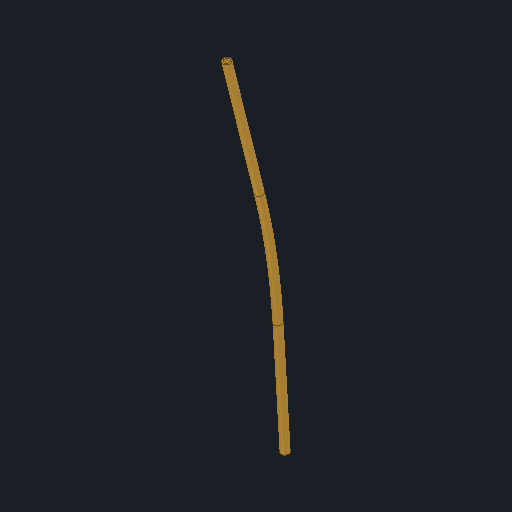
# Autodesk Inventor part: prop_shaft
Saved by Autodesk Inventor 2023 (Build 270158030, 158C)
## iProperties
Created: 2022-04-18
Part Number: prop_shaft
Material: Generic
Document SubType Name: Modeling
Designer: kardo
Density: 1 g/cm^3
Appearance: Brass - Prop shaft
Author: kardo
Autodesk Inventor part; units mm, degrees
ref_plane "YZ Plane" through (0, 0, 0) normal (1, 0, 0) x (0, 1, 0)
ref_plane "XZ Plane" through (0, 0, 0) normal (0, 1, 0) x (-1, 0, 0)
ref_plane "XY Plane" through (0, 0, 0) normal (0, 0, 1) x (1, 0, 0)
derived "stencil_frame.ipt"
sketch "sk_drivetrain_profile" plane through (6, 0, 0) normal (1, 0, 0) x (0, 1, 0)
  line L0 (-547.3485, 0) -> (393.091, 0) construction
  line L1 (-363, 4666.1952) -> (-363, -2045.0469) construction
  line L2 (0, 4666.1952) -> (0, -2045.0469) construction
  line L3 (-140.6277, 54.4571) -> (-133.8539, 27.2888)
  line L4 (-395, 0) -> (-331.1194, 3.9071)
  line L5 (-137.2408, 40.8729) -> (-228.5101, 18.117)
  line L6 (-314.0499, 4.9511) -> (-270.6751, 7.604) construction
  line L7 (-270.6751, 7.604) -> (-228.5101, 18.117) construction
  line L8 (-133.8539, 27.2888) -> (-133.8539, 22.2888) construction
  line L9 (-331.1194, 3.9071) -> (-314.0499, 4.9511)
  line L10 (-1246.9714, 4491.7596) -> (383.4376, -2047.4538) construction
  line L11 (-229.1821, 20.8126) -> (-137.9129, 43.5685) construction
  line L12 (-136.5687, 38.1773) -> (-227.838, 15.4214) construction
  line L13 (-229.1821, 20.8126) -> (-227.838, 15.4214) construction
  spline S0 degree 2 poles (-314.0499, 4.9511) (-270.6751, 7.604) (-228.5101, 18.117) knots 1 1 1 2 2 2
  line L14 (0, 21.4767) -> (-254.1001, 20.7404) construction
  line L15 (-55.6943, 22.5153) -> (-309.842, 21.7788) construction
  point P0 (0, 0)
  point P1 (-217.5636, 20.8462)
  point P2 (-205.945, 20.8799)
  point P3 (-201.0754, 22.094)
ref_plane "plane_motor_mount" through (0, -127.05, 0) normal (0, 0.9702957, 0.2419219) x (-1, 0, 0)
sketch "sk_prop_shaft_profile" plane through (0, -127.05, 0) normal (0, 0.9702957, 0.2419219) x (-1, 0, 0)
  circle A0 centre (-6, 42.1242) radius 2.7781
  point P0 (0, -30.7362)
  dimension "d1" = 5.5563
  constraints: 1 centre point, 1 coincident
  measures "d1" diameter of A0
derived "parameters_powertrain.ipt"
sweep "Sweep1" add profiles "sk_prop_shaft_profile" path "sk_drivetrain_profile" path curves L5 S0 L9 L4
shell "Shell1" thickness 0.7937 removed faces 2 at (6.8991, -395.0135, 0.2212) at (6.6932, -137.3893, 41.4688)
equation "\"d1\" = prop_shaft_sleeve_od"
equation "\"prop_shaft_sleeve_od\" = 5.55625"
body "Solid1"
